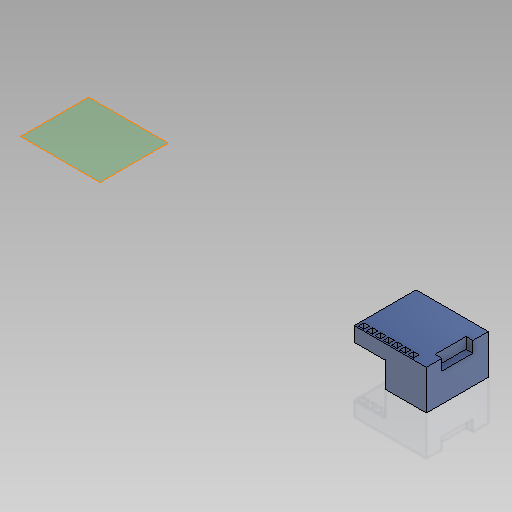
# Autodesk Inventor part: ЛЦМК0000002.00.00.00.00.04
Saved by Autodesk Inventor 2021.2 (Build 252289000, 289)
## iProperties
Created: 2025-10-23
Part Number: ЛЦМК0000002.00.00.00.00.04
Material: Типовые
Document SubType Name: Modeling
Designer: Захаров
Density: 1 g/cm^3
Appearance: С вкраплениями — сатинированная — синяя
Author: Захаров
Autodesk Inventor part; units mm, degrees
ref_plane "YZ Plane" through (0, 0, 0) normal (1, 0, 0) x (0, 1, 0)
ref_plane "XZ Plane" through (0, 0, 0) normal (0, 1, 0) x (-1, 0, 0)
ref_plane "XY Plane" through (0, 0, 0) normal (0, 0, 1) x (1, 0, 0)
ref_plane "РабПлоскость1" through (104.25, -2.8, -7.7) normal (0, -1, 0) x (1, 0, 0)
sketch "Эскиз1" plane through (104.25, -2.8, -7.7) normal (0, -1, 0) x (1, 0, 0)
  line L0 (91.65, 6.9) -> (90.05, 6.9) projected
  line L1 (90.05, 6.9) -> (90.05, 8.5) projected
  line L2 (90.05, 8.5) -> (91.65, 8.5) projected
  line L3 (91.65, 8.5) -> (91.65, 6.9) projected
  line L4 (86.85, 6.9) -> (85.25, 6.9) projected
  line L5 (85.25, 6.9) -> (85.25, 8.5) projected
  line L6 (85.25, 8.5) -> (86.85, 8.5) projected
  line L7 (86.85, 8.5) -> (86.85, 6.9) projected
  line L8 (96.45, 6.9) -> (94.85, 6.9) projected
  line L9 (94.85, 6.9) -> (94.85, 8.5) projected
  line L10 (94.85, 8.5) -> (96.45, 8.5) projected
  line L11 (96.45, 8.5) -> (96.45, 6.9) projected
  line L12 (94.05, 6.9) -> (92.45, 6.9) projected
  line L13 (92.45, 6.9) -> (92.45, 8.5) projected
  line L14 (92.45, 8.5) -> (94.05, 8.5) projected
  line L15 (94.05, 8.5) -> (94.05, 6.9) projected
  line L16 (98.85, 6.9) -> (97.25, 6.9) projected
  line L17 (97.25, 6.9) -> (97.25, 8.5) projected
  line L18 (97.25, 8.5) -> (98.85, 8.5) projected
  line L19 (98.85, 8.5) -> (98.85, 6.9) projected
  line L20 (89.25, 6.9) -> (87.65, 6.9) projected
  line L21 (87.65, 6.9) -> (87.65, 8.5) projected
  line L22 (87.65, 8.5) -> (89.25, 8.5) projected
  line L23 (89.25, 8.5) -> (89.25, 6.9) projected
  line L24 (101.25, 6.9) -> (99.65, 6.9) projected
  line L25 (99.65, 6.9) -> (99.65, 8.5) projected
  line L26 (99.65, 8.5) -> (101.25, 8.5) projected
  line L27 (101.25, 8.5) -> (101.25, 6.9) projected
  line L28 (103.5, 4.5) -> (105.5, 4.5) projected
  line L29 (105.5, 4.5) -> (105.5, 9) projected
  line L30 (105.5, 9) -> (84.5, 9) projected
  line L31 (84.5, 9) -> (84.5, -9) projected
  line L32 (84.5, -9) -> (105.5, -9) projected
  line L33 (105.5, -9) -> (105.5, -4.5) projected
  line L34 (105.5, -4.5) -> (103.5, -4.5) projected
  line L35 (103.5, -4.5) -> (103.5, 4.5) projected
  line L36 (90.05, -6.9) -> (91.65, -6.9) projected
  line L37 (91.65, -6.9) -> (91.65, -8.5) projected
  line L38 (91.65, -8.5) -> (90.05, -8.5) projected
  line L39 (90.05, -8.5) -> (90.05, -6.9) projected
  line L40 (85.25, -6.9) -> (86.85, -6.9) projected
  line L41 (86.85, -6.9) -> (86.85, -8.5) projected
  line L42 (86.85, -8.5) -> (85.25, -8.5) projected
  line L43 (85.25, -8.5) -> (85.25, -6.9) projected
  line L44 (94.85, -6.9) -> (96.45, -6.9) projected
  line L45 (96.45, -6.9) -> (96.45, -8.5) projected
  line L46 (96.45, -8.5) -> (94.85, -8.5) projected
  line L47 (94.85, -8.5) -> (94.85, -6.9) projected
  line L48 (92.45, -6.9) -> (94.05, -6.9) projected
  line L49 (94.05, -6.9) -> (94.05, -8.5) projected
  line L50 (94.05, -8.5) -> (92.45, -8.5) projected
  line L51 (92.45, -8.5) -> (92.45, -6.9) projected
  line L52 (97.25, -6.9) -> (98.85, -6.9) projected
  line L53 (98.85, -6.9) -> (98.85, -8.5) projected
  line L54 (98.85, -8.5) -> (97.25, -8.5) projected
  line L55 (97.25, -8.5) -> (97.25, -6.9) projected
  line L56 (87.65, -6.9) -> (89.25, -6.9) projected
  line L57 (89.25, -6.9) -> (89.25, -8.5) projected
  line L58 (89.25, -8.5) -> (87.65, -8.5) projected
  line L59 (87.65, -8.5) -> (87.65, -6.9) projected
  line L60 (99.65, -6.9) -> (101.25, -6.9) projected
  line L61 (101.25, -6.9) -> (101.25, -8.5) projected
  line L62 (101.25, -8.5) -> (99.65, -8.5) projected
  line L63 (99.65, -8.5) -> (99.65, -6.9) projected
  point P0 (-104.25, 7.7)
extrude "Выдавливание1" add sketch "Эскиз1" along normal blind 4.2 contours L35 L34 L33 L32 L31 L30 L29 L28 | L36 L37 L38 L39 | L40 L41 L42 L43 | L44 L45 L46 L47 | L48 L49 L50 L51 | L52 L53 L54 L55 | L56 L57 L58 L59 | L60 L61 L62 L63
sketch "Эскиз2" plane through (104.25, -7, -7.7) normal (0, -1, 0) x (1, 0, 0)
  line L0 (105.5, -9) -> (105.5, -4.5) projected
  line L1 (105.5, 9) -> (84.5, 9) projected
  line L2 (105.5, -9) -> (93.5, -9)
  line L3 (93.5, -9) -> (93.5, 9)
  line L4 (93.5, 9) -> (105.5, 9)
  line L5 (105.5, 9) -> (105.5, -9)
  point P0 (-104.25, 7.7)
  point P1 (105.5, 9)
  dimension "d2" = 12
  constraints: 8 end point, 2 parallel, 1 horizontal, 1 perpendicular, 1 point on line
  measures "d2" distance of L3.end L4.end
extrude "Выдавливание2" add sketch "Эскиз2" along normal blind 7.3
sketch "Эскиз3" plane through (104.25, -14.3, -7.7) normal (0, -1, 0) x (1, 0, 0)
  line L0 (90.05, 6.9) -> (91.65, 6.9) projected
  line L1 (91.65, 6.9) -> (91.65, 8.5) projected
  line L2 (91.65, 8.5) -> (90.05, 8.5) projected
  line L3 (90.05, 8.5) -> (90.05, 6.9) projected
  line L4 (85.25, 6.9) -> (86.85, 6.9) projected
  line L5 (86.85, 6.9) -> (86.85, 8.5) projected
  line L6 (86.85, 8.5) -> (85.25, 8.5) projected
  line L7 (85.25, 8.5) -> (85.25, 6.9) projected
  line L8 (94.85, 6.9) -> (96.45, 6.9) projected
  line L9 (96.45, 6.9) -> (96.45, 8.5) projected
  line L10 (96.45, 8.5) -> (94.85, 8.5) projected
  line L11 (94.85, 8.5) -> (94.85, 6.9) projected
  line L12 (92.45, 6.9) -> (94.05, 6.9) projected
  line L13 (94.05, 6.9) -> (94.05, 8.5) projected
  line L14 (94.05, 8.5) -> (92.45, 8.5) projected
  line L15 (92.45, 8.5) -> (92.45, 6.9) projected
  line L16 (97.25, 6.9) -> (98.85, 6.9) projected
  line L17 (98.85, 6.9) -> (98.85, 8.5) projected
  line L18 (98.85, 8.5) -> (97.25, 8.5) projected
  line L19 (97.25, 8.5) -> (97.25, 6.9) projected
  line L20 (87.65, 6.9) -> (89.25, 6.9) projected
  line L21 (89.25, 6.9) -> (89.25, 8.5) projected
  line L22 (89.25, 8.5) -> (87.65, 8.5) projected
  line L23 (87.65, 8.5) -> (87.65, 6.9) projected
  line L24 (99.65, 6.9) -> (101.25, 6.9) projected
  line L25 (101.25, 6.9) -> (101.25, 8.5) projected
  line L26 (101.25, 8.5) -> (99.65, 8.5) projected
  line L27 (99.65, 8.5) -> (99.65, 6.9) projected
  line L28 (105.5, 9) -> (84.5, 9) projected
  line L29 (105.5, -9) -> (105.5, 9) projected
  line L30 (84.5, -9) -> (105.5, -9) projected
  line L31 (84.5, 9) -> (84.5, -9) projected
  line L32 (91.65, -6.9) -> (90.05, -6.9) projected
  line L33 (90.05, -6.9) -> (90.05, -8.5) projected
  line L34 (90.05, -8.5) -> (91.65, -8.5) projected
  line L35 (91.65, -8.5) -> (91.65, -6.9) projected
  line L36 (86.85, -6.9) -> (85.25, -6.9) projected
  line L37 (85.25, -6.9) -> (85.25, -8.5) projected
  line L38 (85.25, -8.5) -> (86.85, -8.5) projected
  line L39 (86.85, -8.5) -> (86.85, -6.9) projected
  line L40 (96.45, -6.9) -> (94.85, -6.9) projected
  line L41 (94.85, -6.9) -> (94.85, -8.5) projected
  line L42 (94.85, -8.5) -> (96.45, -8.5) projected
  line L43 (96.45, -8.5) -> (96.45, -6.9) projected
  line L44 (94.05, -6.9) -> (92.45, -6.9) projected
  line L45 (92.45, -6.9) -> (92.45, -8.5) projected
  line L46 (92.45, -8.5) -> (94.05, -8.5) projected
  line L47 (94.05, -8.5) -> (94.05, -6.9) projected
  line L48 (98.85, -6.9) -> (97.25, -6.9) projected
  line L49 (97.25, -6.9) -> (97.25, -8.5) projected
  line L50 (97.25, -8.5) -> (98.85, -8.5) projected
  line L51 (98.85, -8.5) -> (98.85, -6.9) projected
  line L52 (89.25, -6.9) -> (87.65, -6.9) projected
  line L53 (87.65, -6.9) -> (87.65, -8.5) projected
  line L54 (87.65, -8.5) -> (89.25, -8.5) projected
  line L55 (89.25, -8.5) -> (89.25, -6.9) projected
  line L56 (101.25, -6.9) -> (99.65, -6.9) projected
  line L57 (99.65, -6.9) -> (99.65, -8.5) projected
  line L58 (99.65, -8.5) -> (101.25, -8.5) projected
  line L59 (101.25, -8.5) -> (101.25, -6.9) projected
  point P0 (-104.25, 7.7)
extrude "Выдавливание3" cut sketch "Эскиз3" against normal blind 7.3 contours L11 L10 L9 L8 | L15 L14 L13 L12 | L19 L18 L17 L16 | L27 L26 L25 L24
sketch "Эскиз4" plane through (104.25, -7, -7.7) normal (0, 1, 0) x (1, 0, 0)
  line L0 (103.5, -4.5) -> (105.5, -4.5) projected
  line L1 (105.5, 4.5) -> (105.5, -4.5) projected
  line L2 (105.5, 4.5) -> (103.5, 4.5) projected
  line L3 (103.5, 4.5) -> (103.5, -4.5) projected
  point P0 (-104.25, -7.7)
ref_plane "РабПлоскость2" through (10.25, -6, -12.2) normal (0, -1, 0) x (1, 0, 0)
extrude "Выдавливание4" add sketch "Эскиз4" along normal up to surface (1 mm away)
